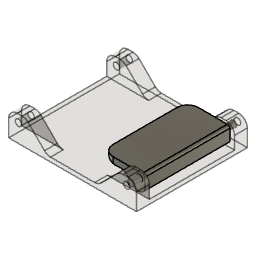
ACUTE_Klemma v1 (Autodesk Fusion 360 design; units mm, degrees)
Autodesk Fusion 360 part; units mm, degrees
sketch "Sketch1" plane through (0, 0, 0) normal (0, 0, 1) x (1, 0, 0)
  line L0 (0, 0) -> (30, 0)
  line L1 (30, 0) -> (30, 26)
  line L2 (30, 26) -> (0, 26)
  line L3 (0, 26) -> (0, 0)
  dimension "d1" = 30
  dimension "d2" = 26
  constraint horizontal L0
  constraint vertical L1
  constraint horizontal L2
  constraint vertical L3
  constraint coincident L0.start L3.end
  measures "d1" distance of L0.start L0.end
  measures "d2" distance of L0.start L2.end
extrude "Extrude1" add sketch "Sketch1" along normal blind 6 makes body 1
sketch "Sketch2" plane through (0, 0, 0) normal (0, -1, 0) x (1, 0, 0)
  line L0 (0, 0) -> (30, 0)
  line L1 (30, 0) -> (30, 6)
  line L2 (30, 6) -> (0, 6)
  line L3 (0, 6) -> (0, 0)
  line L4 (0, 0) -> (0, 4) construction
  line L5 (0, 6) -> (2, 6) construction
  arc A0 (2, 6) -> (0, 4) centre (2, 4) ccw
  line L6 (2, 6) -> (3.1716, 6)
  line L7 (0, 0) -> (0, 1) construction
  line L8 (0, 1) -> (30, 1) construction
  line L9 (4.5858, 5.4142) -> (8.4142, 1.5858)
  line L10 (4, 6) -> (11.0711, 6) construction
  line L11 (15, 6) -> (15, 0) construction
  line L12 (25.4142, 5.4142) -> (21.5858, 1.5858)
  arc A1 (30, 4) -> (28, 6) centre (28, 4) ccw
  line L13 (28, 6) -> (26.8284, 6)
  line L14 (9.8284, 1) -> (20.1716, 1)
  arc A2 (26.8284, 6) -> (25.4142, 5.4142) centre (26.8284, 4) ccw
  arc A3 (4.5858, 5.4142) -> (3.1716, 6) centre (3.1716, 4) ccw
  arc A4 (8.4142, 1.5858) -> (9.8284, 1) centre (9.8284, 3) ccw
  arc A5 (20.1716, 1) -> (21.5858, 1.5858) centre (20.1716, 3) ccw
  dimension "d5" = 4
  dimension "d6" = 2
  dimension "d7" = 2
  dimension "d8" = 1
  dimension "d9" = 45
  dimension "d10" = 2
  dimension "d11" = 2
  constraint coincident L0.start L3.end
  constraint perpendicular L2 L4
  constraint coincident L2.end L3.start
  constraint perpendicular L3 L5
  constraint tangent L5 A0
  constraint parallel L2 L6
  constraint parallel L4 L7
  constraint coincident L1 L8.end
  constraint perpendicular L1 L8
  constraint horizontal L10
  constraint midpoint L2 L11.start
  constraint midpoint L0 L11.end
  constraint symmetric L4.end L11 A1.start
  constraint symmetric L5.end L11 A1.end
  constraint symmetric A0 L11 A1
  constraint tangent L12 A2
  constraint tangent L13 A2
  constraint coincident L10.start L9
  constraint coincident L10.start L6
  constraint tangent L9 A3
  constraint tangent L6 A3
  constraint equal A2 A3
  constraint tangent L9 A4
  constraint tangent L14 A4
  constraint tangent L12 A5
  constraint tangent L14 A5
  constraint equal A4 A5
  measures "d5" distance of L0.start L4.end
  measures "d6" distance of L2.end L5.end
  measures "d7" distance of L5.end L10.start
  measures "d8" distance of L0.start L7.end
  measures "d9" angle of L9 L10
  measures "d10" radius of A2
  measures "d11" radius of A4
extrude "Extrude2" cut sketch "Sketch2" against normal blind 27 contours L2 L3 A0 | L1 L2 A1 | L2 L9 L12 L14 A2 A3 A4 A5 bodies 1
sketch "Sketch3" plane through (30, 0, 0) normal (1, 0, 0) x (0, 1, 0)
  line L0 (26, 4) -> (0, 4)
  line L1 (0, 4) -> (0, 0)
  line L2 (0, 0) -> (26, 0)
  line L3 (26, 0) -> (26, 4)
  line L4 (26, 6) -> (0, 6)
  line L5 (0, 6) -> (0, 4) construction
  line L6 (0, 4) -> (26, 4) construction
  line L7 (26, 4) -> (26, 6)
  line L8 (0, 6) -> (3, 6) construction
  line L9 (26, 6) -> (23, 6) construction
  line L10 (3, 6) -> (3, 1)
  line L11 (23, 6) -> (23, 1)
  line L12 (23, 1) -> (3, 1)
  dimension "d14" = 3
  dimension "d15" = 3
  dimension "d16" = 5
  dimension "d17" = 5
  constraint coincident L4.end L5.start
  constraint perpendicular L5 L8
  constraint coincident L4.start L7.end
  constraint perpendicular L7 L9
  constraint perpendicular L2 L10
  constraint perpendicular L6 L11
  measures "d14" distance of L4.end L8.end
  measures "d15" distance of L4.start L9.end
  measures "d16" distance of L8.end L10.end
  measures "d17" distance of L9.end L11.end
extrude "Extrude3" cut sketch "Sketch3" against normal blind 33 contours L0 L10 L11 L12 | L0 L4 L10 L11 bodies 1
sketch "Sketch4" plane through (0, 26, 0) normal (0, 1, 0) x (-1, 0, 0)
  arc A0 (-28, 6) -> (-30, 4) centre (-28, 4) ccw
  line L0 (-30, 4) -> (-30, 0)
  line L1 (-30, 0) -> (0, 0)
  line L2 (0, 0) -> (0, 4)
  arc A1 (0, 4) -> (-2, 6) centre (-2, 4) ccw
  line L3 (-2, 6) -> (-3.1716, 6)
  arc A2 (-3.1716, 6) -> (-4.5858, 5.4142) centre (-3.1716, 4) ccw
  line L4 (-4.5858, 5.4142) -> (-8.4142, 1.5858)
  arc A3 (-9.8284, 1) -> (-8.4142, 1.5858) centre (-9.8284, 3) ccw
  line L5 (-9.8284, 1) -> (-20.1716, 1)
  arc A4 (-21.5858, 1.5858) -> (-20.1716, 1) centre (-20.1716, 3) ccw
  line L6 (-21.5858, 1.5858) -> (-25.4142, 5.4142)
  arc A5 (-25.4142, 5.4142) -> (-26.8284, 6) centre (-26.8284, 4) ccw
  line L7 (-26.8284, 6) -> (-28, 6)
  line L8 (0, 0) -> (0, 3) construction
  line L9 (0, 3) -> (-4.5858, 5.4142) construction
  circle A6 centre (-2.2929, 4.2071) radius 0.75
  line L10 (-30, 0) -> (-30, 3) construction
  line L11 (-30, 3) -> (-25.4142, 5.4142) construction
  circle A7 centre (-27.7071, 4.2071) radius 0.75
  dimension "d22" = 3
  dimension "d23" = 1.5
  dimension "d24" = 3
  dimension "d25" = 1.5
  constraint coincident L1.end L2.start
  constraint perpendicular L1 L8
  constraint coincident A2.end L4.start
  constraint midpoint L9 A6.centre
  constraint coincident L0.end L1.start
  constraint perpendicular L1 L10
  constraint coincident L6.end A5.start
  constraint midpoint L11 A7.centre
  measures "d22" distance of L1.end L8.end
  measures "d23" diameter of A6
  measures "d24" distance of L0.end L10.end
  measures "d25" diameter of A7
extrude "Extrude4" cut sketch "Sketch4" against normal blind 40 contours A6 | A7 bodies 1
sketch "Sketch5" plane through (0, 0, 0) normal (-1, 0, 0) x (0, -1, 0)
  line L0 (-3, 4) -> (-3, 1)
  line L1 (-3, 1) -> (-23, 1)
  line L2 (-23, 1) -> (-23, 4)
  line L3 (-23, 4) -> (-26, 4)
  line L4 (-26, 4) -> (-26, 0)
  line L5 (-26, 0) -> (0, 0)
  line L6 (0, 0) -> (0, 4)
  line L7 (0, 4) -> (-3, 4)
  line L8 (-23, 1) -> (-3, 1)
  line L9 (-3, 1) -> (-3, 3)
  line L10 (-3, 3) -> (-23, 3)
  line L11 (-23, 3) -> (-23, 1)
  dimension "d28" = 2
  constraint horizontal L8
  constraint vertical L9
  constraint horizontal L10
  constraint vertical L11
  constraint coincident L1.end L2.start
  measures "d28" distance of L1.end L10.end
extrude "Extrude5" add sketch "Sketch5" along normal blind 17 and the other way blind 47 separate body contours L0 L1 L2 L8 L9 L10 L11 makes body 2
sketch "Sketch6" plane through (0, 23, 0) normal (0, -1, 0) x (1, 0, 0)
  circle A0 centre (27.7071, 4.2071) radius 0.75
  arc A1 (30, 4) -> (28, 6) centre (28, 4) ccw
  line L0 (28, 6) -> (26.8284, 6)
  arc A2 (26.8284, 6) -> (25.4142, 5.4142) centre (26.8284, 4) ccw
  line L1 (25.4142, 5.4142) -> (21.5858, 1.5858)
  arc A3 (20.1716, 1) -> (21.5858, 1.5858) centre (20.1716, 3) ccw
  line L2 (20.1716, 1) -> (30, 1)
  line L3 (30, 1) -> (30, 4)
  circle A4 centre (27.7071, 4.2071) radius 0.75 construction
  circle A5 centre (2.2929, 4.2071) radius 0.75 construction
  arc A6 (30, 4) -> (28, 6) centre (28, 4) ccw construction
  line L4 (28, 6) -> (26.8284, 6) construction
  arc A7 (26.8284, 6) -> (25.4142, 5.4142) centre (26.8284, 4) ccw construction
  line L5 (25.4142, 5.4142) -> (21.5858, 1.5858) construction
  arc A8 (20.1716, 1) -> (21.5858, 1.5858) centre (20.1716, 3) ccw construction
  line L6 (20.1716, 1) -> (9.8284, 1) construction
  arc A9 (8.4142, 1.5858) -> (9.8284, 1) centre (9.8284, 3) ccw construction
  line L7 (8.4142, 1.5858) -> (4.5858, 5.4142) construction
  arc A10 (4.5858, 5.4142) -> (3.1716, 6) centre (3.1716, 4) ccw construction
  line L8 (3.1716, 6) -> (2, 6) construction
  arc A11 (2, 6) -> (0, 4) centre (2, 4) ccw construction
  line L9 (0, 4) -> (0, 0) construction
  line L10 (0, 0) -> (30, 0) construction
  line L11 (30, 0) -> (30, 4) construction
  line L12 (47, 3) -> (-17, 3) construction
  line L13 (-17, 3) -> (-17, 1) construction
  line L14 (-17, 1) -> (47, 1) construction
  line L15 (47, 1) -> (47, 3) construction
  circle A12 centre (27.7071, 4.2071) radius 0.725
  line L16 (27.7071, 4.2071) -> (27.7071, 1.4071) construction
  line L17 (28.9197, 2.1921) -> (25.9056, 2.1921) construction
  line L18 (25.9056, 2.1921) -> (24, 4)
  line L19 (25.4142, 5.4142) -> (15, 5.4142)
  line L20 (15, 5.4142) -> (15, 4)
  line L21 (15, 4) -> (24, 4)
  line L22 (28.9197, 2.1921) -> (28.9197, 4.9423)
  arc A13 (28.9197, 4.1897) -> (28.9197, 2.1921) centre (27.4127, 3.1909) ccw
  line L23 (25.4142, 5.4142) -> (28.2984, 5.4142)
  arc A14 (28.9197, 4.9423) -> (28.2984, 5.4142) centre (28.2984, 4.7692) ccw
  dimension "d33" = 1.45
  dimension "d34" = 2.8
  constraint concentric A4 A12
  constraint coincident A0.centre A4.centre
  constraint perpendicular L12 L16
  constraint tangent A4 A13
  constraint coincident L16.end A13
  constraint coincident L17.end A13
  constraint parallel L12 L17
  constraint coincident L5 L18.end
  constraint coincident A2.end L1.start
  constraint parallel L12 L19
  constraint perpendicular L19 L20
  constraint perpendicular L20 L21
  constraint perpendicular L17 L22
  constraint coincident L22 A13.start
  constraint perpendicular L22 L23
  constraint tangent L23 A14
  measures "d33" diameter of A12
  measures "d34" distance of A0.centre L16.end
extrude "Extrude6" add sketch "Sketch6" along normal blind 20 separate body contours A0 | L22 A13 | L1 L18 L22 A13 L23 A14 | L1 L19 L20 L21 | A12 makes body 3
extrude "Extrude7" add sketch "Sketch6" along normal blind 22 and the other way blind 2 contours A12 bodies 3
extrude "Extrude8" cut 1 faces at (15, 16.3333, 4.9428) along direction (1, 0, 0) blind 4 on bodies 3 bodies 3
chamfer "Chamfer1" distance 2.5 distance2 1 2 edges at (19, 13, 4) (25.9056, 13, 2.1921) measured on face at (20.6667, 16.3333, 4) measured on face at (25.2704, 9.6667, 2.7948) on bodies 3
fillet "Fillet1" radius 2.5 2 edges at (19, 3, 5.2071) (19, 23, 5.2071) on bodies 3
hidden bodies 2
